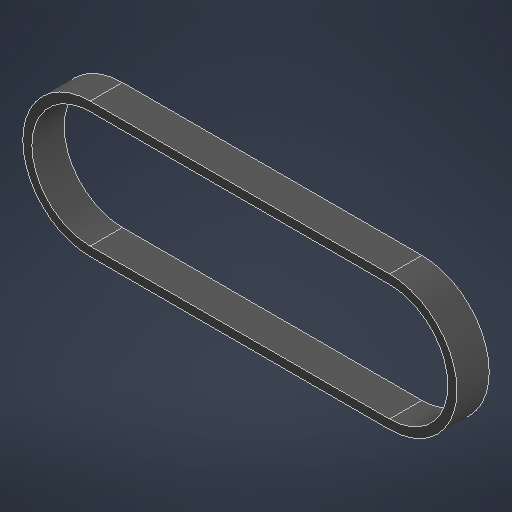
# Autodesk Inventor part: 55t_Belt
Saved by Autodesk Inventor 2026.2 (Build 302298010, 298A)
## iProperties
Created: 2026-04-01
Part Number: 55t_Belt
Material: Rubber
Document SubType Name: Modeling
Designer: 4aida
Density: 0.93 g/cm^3
Appearance: Generic
Author: 4aida
Autodesk Inventor part; units mm, degrees
ref_plane "YZ Plane" through (0, 0, 0) normal (1, 0, 0) x (0, 1, 0)
ref_plane "XZ Plane" through (0, 0, 0) normal (0, 1, 0) x (-1, 0, 0)
ref_plane "XY Plane" through (0, 0, 0) normal (0, 0, 1) x (1, 0, 0)
sketch "Sketch1" plane through (0, 0, 0) normal (1, 0, 0) x (0, 1, 0)
  line L0 (1.27, -4.5) -> (-1.27, -4.5)
  line L1 (-1.27, -4.5) -> (-1.27, 4.5)
  line L2 (-1.27, 4.5) -> (1.27, 4.5)
  line L3 (1.27, 4.5) -> (1.27, -4.5)
  line L4 (1.27, -4.5) -> (-1.27, 4.5) construction
  line L5 (-1.27, -4.5) -> (1.27, 4.5) construction
  point P0 (0, 0)
  point P1 (0, 0)
  dimension "d0" = 9
  dimension "d1" = 2.54
  constraints: 12 end point, 2 midpoint, 2 parallel, 1 coincident, 1 horizontal, 1 perpendicular
  measures "d0" distance of L2.end L0.start
  measures "d1" distance of L1.end L2.end
sketch "Sketch2" plane through (0, 0, 0) normal (0, 0, 1) x (1, 0, 0)
  arc A0 (-41.75, 0) -> (-41.75, -35.0141) centre (-41.75, -17.507) ccw
  arc A1 (41.75, -35.0141) -> (41.75, 0) centre (41.75, -17.507) ccw
  line L0 (-41.75, 0) -> (41.75, 0)
  line L1 (41.75, -35.0141) -> (-41.75, -35.0141)
  point P0 (0, 0)
  point P1 (0, 0)
  dimension "d2" = 83.5
  dimension "d3" = 17.507
  constraints: 4 end point, 4 point on circle, 4 tangent, 2 centre point, 2 horizontal, 1 coincident, 1 midpoint
  measures "d2" distance of A1.centre A0.centre
  measures "d3" radius of A0
sweep "Sweep1" add profiles "Sketch1" path "Sketch2"
body "Solid1"
